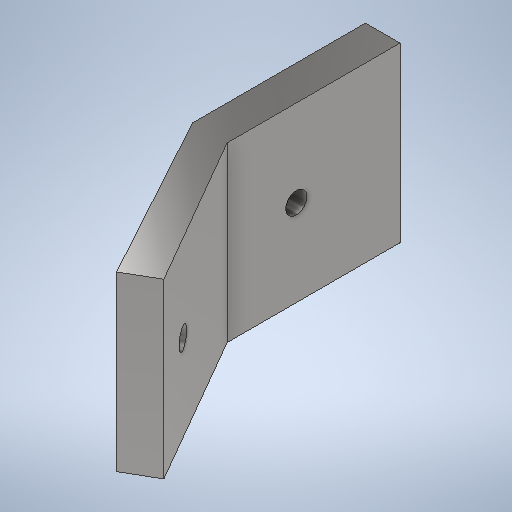
# Autodesk Inventor part: 150degreebracket
Saved by Autodesk Inventor 2025.2 (Build 292293000, 293)
## iProperties
Created: 2026-03-19
Part Number: 150degreebracket
Material: Iron, Malleable
Document SubType Name: Modeling
Designer: hp
Density: 7.15 g/cm^3
Appearance: Semi-Polished
Author: hp
Autodesk Inventor part; units mm, degrees
ref_plane "YZ Plane" through (0, 0, 0) normal (1, 0, 0) x (0, 1, 0)
ref_plane "XZ Plane" through (0, 0, 0) normal (0, 1, 0) x (-1, 0, 0)
ref_plane "XY Plane" through (0, 0, 0) normal (0, 0, 1) x (1, 0, 0)
sketch "Sketch1" plane through (0, 0, 0) normal (0, 1, 0) x (-1, 0, 0)
  line L0 (0, 0) -> (4, 0)
  line L1 (4, 0) -> (4, -20)
  line L2 (4, -20) -> (0, -20)
  line L3 (0, -20) -> (0, 0)
  line L4 (0, 0) -> (-10, 17.3205)
  line L5 (0, 0) -> (20, 0) construction
  line L6 (-10, 17.3205) -> (-6.5359, 19.3205)
  line L7 (-6.5359, 19.3205) -> (4, 0)
  dimension "d0" = 4
  dimension "d1" = 20
  dimension "d2" = 20
  dimension "d3" = 120
  dimension "d4" = 4
  constraints: 16 end point, 2 horizontal, 2 parallel, 2 perpendicular, 1 equal length
  measures "d0" distance of L1.end L2.end
  measures "d1" distance of L0.end L1.end
  measures "d2" distance of L0.start L4.end
  measures "d3" angle of L5 L4
  measures "d4" distance of L4.end L6.end
extrude "Extrusion1" add sketch "Sketch1" along normal blind 20
sketch "Sketch2" plane through (0, 0, 0) normal (1, 0, 0) x (0, 0, -1)
  line L0 (0, 0) -> (0, 20) projected
  line L1 (0, 0) -> (20, 0) projected
  point P0 (8, 10)
  point P1 (0, 10)
  dimension "d7" = 8
  dimension "d8" = 10
  constraints: 1 midpoint
  measures "d7" distance of point (8, 10) point (0, 10)
  measures "d8" distance from line of L1 point (8, 10)
hole "Hole1" at (0, 10, -8) direction (-1, 0, 0) diameter 2.45 end through all
sketch "Sketch3" plane through (0, 0, 0) normal (0.8660254, 0, -0.5) x (-0.5, 0, -0.8660254)
  line L0 (0, 0) -> (0, 20) projected
  line L1 (-20, 20) -> (0, 20) projected
  point P0 (-14, 10)
  point P1 (0, 10)
  dimension "d16" = 14
  dimension "d17" = 10
  constraints: 1 midpoint
  measures "d16" distance of point (0, 10) point (-14, 10)
  measures "d17" distance from line of point (-14, 10) L1
hole "Hole2" at (7, 10, 12.1244) direction (-0.8660254, 0, 0.5) diameter 2.45 end through all
equation "\"d0\" = d4"
body "Solid1"
